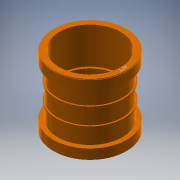
# Autodesk Inventor part: doubleSocketPipe
Saved by Autodesk Inventor 2016 (Build 200138000, 138)
## iProperties
Created: 2015-11-22
Part Number: doubleSocketPipe
Material: PVC-Piping
Document SubType Name: Modeling
Designer: Artur
Density: 1.4 g/cm^3
Appearance: Smooth - White
Author: Artur
Autodesk Inventor part; units mm, degrees
ref_plane "YZ Plane" through (0, 0, 0) normal (1, 0, 0) x (0, 1, 0)
ref_plane "XZ Plane" through (0, 0, 0) normal (0, 1, 0) x (-1, 0, 0)
ref_plane "XY Plane" through (0, 0, 0) normal (0, 0, 1) x (1, 0, 0)
sketch "Sketch1" plane through (0, 0, 0) normal (1, 0, 0) x (0, 1, 0)
  line L0 (0, 0) -> (0, -141.6259) construction
  line L1 (-13.3, 0) -> (79.8, 0) construction
  line L2 (55.5, -66.5) -> (25.7904, -66.5) construction
  line L3 (51.5, -66) -> (51.5, -67)
  line L4 (51.5, -66) -> (55.5, -66)
  line L5 (55.5, -66) -> (55.5, 0)
  line L6 (51.5, -67) -> (55.5, -67)
  line L7 (55.5, -67) -> (55.5, -127)
  line L8 (66.5, -108.5) -> (58.5, -108.5)
  line L9 (58.5, -108.5) -> (58.5, -80.5)
  line L10 (58.5, -80.5) -> (61, -80.5)
  line L11 (61, -80.5) -> (61, -77.5)
  line L12 (61, -77.5) -> (58.5, -77.5)
  line L13 (58.5, -77.5) -> (58.5, -49.5)
  line L14 (58.5, -49.5) -> (61, -49.5)
  line L15 (61, -49.5) -> (61, -46.5)
  line L16 (61, -46.5) -> (58.5, -46.5)
  line L17 (58.5, -46.5) -> (58.5, -18.5)
  line L18 (58.5, -18.5) -> (66.5, -18.5)
  line L19 (66.5, -18.5) -> (66.5, -1)
  line L20 (66.5, -1) -> (65.5, -1)
  line L21 (65.5, -1) -> (65.5, 0)
  line L22 (65.5, 0) -> (55.5, 0)
  line L23 (66.5, -108.5) -> (66.5, -126)
  line L24 (66.5, -126) -> (65.5, -126)
  line L25 (65.5, -126) -> (65.5, -127)
  line L26 (65.5, -127) -> (55.5, -127)
  point P0 (51.5, -66.5)
  dimension "d2" = 1
  dimension "d3" = 103
  dimension "d4" = 66
  dimension "d5" = 111
  dimension "d6" = 60
  dimension "d9" = 8
  dimension "d10" = 28
  dimension "d11" = 2.5
  dimension "d12" = 3
  dimension "d13" = 28
  dimension "d14" = 2.5
  dimension "d15" = 3
  dimension "d16" = 28
  dimension "d17" = 8
  dimension "d19" = 17.5
  dimension "d20" = 1
  dimension "d21" = 17.5
  dimension "d22" = 1
  dimension "d23" = 3
  dimension "d24" = 1
  dimension "d25" = 1
  constraints: 52 end point, 13 perpendicular, 6 point on line, 4 horizontal, 4 vertical, 2 collinear, 1 midpoint, 1 parallel
  measures "d2" distance of L3.start L3.end
  measures "d3" diameter of L3.end L0
  measures "d4" distance from line of L1 L3.start
  measures "d5" diameter of L5 L0
  measures "d6" distance of L6.end L7.end
  measures "d9" distance of L8.start L8.end
  measures "d10" distance of L8.end L9.end
  measures "d11" distance of L9.end L10.end
  measures "d12" distance of L10.end L11.end
  measures "d13" distance of L12.end L13.end
  measures "d14" distance of L13.end L14.end
  measures "d15" distance of L14.end L15.end
  measures "d16" distance of L16.end L17.end
  measures "d17" distance of L17.end L18.end
  measures "d19" distance of L18.end L19.end
  measures "d20" distance of L19.end L20.end
  measures "d21" distance of L8.start L23.end
  measures "d22" distance of L23.end L24.end
  measures "d23" distance between parallel lines of L7 L9
  measures "d24" distance of L20.end L21.end
  measures "d25" distance of L24.end L25.end
revolve "Revolution1" add sketch "Sketch1" angle 360 about axis through (0, 0, 0) along (0, 0, -1)
sketch "Sketch2" plane through (0, 0, 0) normal (0, 0, 1) x (1, 0, 0)
  line L0 (62.3533, 7.1392) -> (62.3533, -1.0719) construction
  line L1 (62.3533, -1.0719) -> (58.8533, -1.0719) construction
  line L2 (58.8533, -1.0719) -> (58.8533, 7.1392) construction
  line L3 (58.8533, 7.1392) -> (62.3533, 7.1392) construction
  line L4 (56.2533, 7.1788) -> (62.3533, 5.1223)
  line L5 (62.3533, 5.1223) -> (62.3533, 4.1238)
  line L6 (62.3533, 4.1238) -> (56.2533, 2.0674)
  line L7 (56.2533, 2.0674) -> (56.2533, 2.9226)
  line L8 (56.2533, 2.9226) -> (57.9587, 3.4762)
  line L9 (57.9587, 3.4762) -> (57.9587, 5.8045)
  line L10 (57.9587, 5.8045) -> (56.2533, 6.3582)
  line L11 (56.2533, 6.3582) -> (56.2533, 7.1788)
  line L12 (58.6507, 3.6987) -> (61.5228, 4.6429)
  line L13 (61.5228, 4.6429) -> (58.6507, 5.5821)
  line L14 (58.6507, 5.5821) -> (58.6507, 3.6987)
  line L15 (61.6315, -2.1591) -> (61.6315, 0.6783)
  line L16 (61.6315, 0.6783) -> (59.9113, 0.6783)
  line L17 (59.9113, 0.6783) -> (59.9113, -2.0405)
  line L18 (59.9113, -2.0405) -> (59.1896, -2.0405)
  line L19 (59.1896, -2.0405) -> (59.1896, 0.6783)
  line L20 (59.1896, 0.6783) -> (56.2533, 0.6783)
  line L21 (56.2533, 0.6783) -> (56.2533, 1.489)
  line L22 (56.2533, 1.489) -> (62.3533, 1.489)
  line L23 (62.3533, 1.489) -> (62.3533, -2.1591)
  line L24 (62.3533, -2.1591) -> (61.6315, -2.1591)
  line L25 (56.2533, -4.3094) -> (61.6315, -4.3094)
  line L26 (61.6315, -4.3094) -> (61.6315, -2.2629)
  line L27 (61.6315, -2.2629) -> (62.3533, -2.2629)
  line L28 (62.3533, -2.2629) -> (62.3533, -7.1666)
  line L29 (62.3533, -7.1666) -> (61.6315, -7.1666)
  line L30 (61.6315, -7.1666) -> (61.6315, -5.1201)
  line L31 (61.6315, -5.1201) -> (56.2533, -5.1201)
  line L32 (56.2533, -5.1201) -> (56.2533, -4.3094)
  point P0 (0, 0)
  constraints: 2 other
emboss "Emboss1" sketch "Sketch2" operation cut depth 0.001 direction (0, 0, -1)
equation "\"d22\" = d20"
equation "\"d24\" = d20"
equation "\"d25\" = d24"
body "Solid1"
